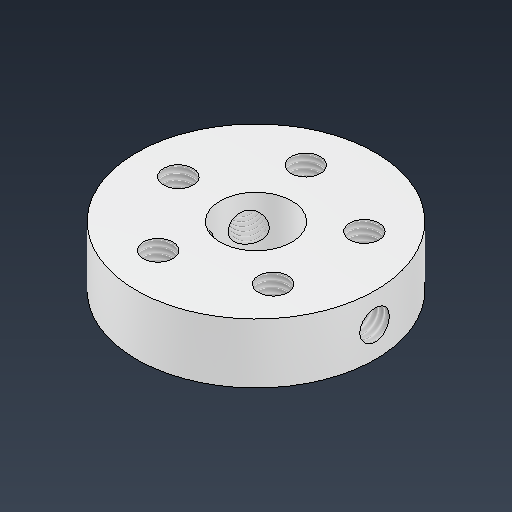
# Autodesk Inventor part: DiyHub
Saved by Autodesk Inventor 2026.2 (Build 302298010, 298A)
## iProperties
Created: 2026-04-20
Part Number: DiyHub
Material: Aluminum 6061
Document SubType Name: Modeling
Designer: szymo
Density: 2.7 g/cm^3
Appearance: Aluminum - Flat
Author: szymo
Autodesk Inventor part; units mm, degrees
ref_plane "YZ Plane" through (0, 0, 0) normal (1, 0, 0) x (0, 1, 0)
ref_plane "XZ Plane" through (0, 0, 0) normal (0, 1, 0) x (-1, 0, 0)
ref_plane "XY Plane" through (0, 0, 0) normal (0, 0, 1) x (1, 0, 0)
sketch "Sketch1" plane through (0, 0, 0) normal (0, 1, 0) x (-1, 0, 0)
  circle A0 centre (0, 0) radius 15 construction
  circle A1 centre (0, 0) radius 10
  circle A2 centre (0, 0) radius 3
  circle A3 centre (0, 0) radius 6.5 construction
  circle A4 centre (6.5, 0) radius 3.25 construction
  line L0 (6.5, 0) -> (0, 0) construction
  circle A5 centre (6.5, 0) radius 1.5 construction
  circle A6 centre (2.0086, 6.1819) radius 1.5 construction
  circle A7 centre (2.0086, 6.1819) radius 3.25 construction
  circle A8 centre (-5.2586, 3.8206) radius 1.5 construction
  circle A9 centre (-5.2586, 3.8206) radius 3.25 construction
  circle A10 centre (-5.2586, -3.8206) radius 1.5 construction
  circle A11 centre (-5.2586, -3.8206) radius 3.25 construction
  circle A12 centre (2.0086, -6.1819) radius 1.5 construction
  circle A13 centre (2.0086, -6.1819) radius 3.25 construction
  dimension "d4" = 13
  dimension "d0" = 30
  dimension "d1" = 5
  dimension "d2" = 20
  dimension "d3" = 6
  dimension "d5" = 6.5
  dimension "d6" = 3
  dimension "d9" = 360
  constraints: 13 centre point, 9 coincident, 2 end point, 1 horizontal, 1 horizontal alignment, 23 other
  measures "d0" diameter of A0
  measures "d1" radial gap between concentric circles of A0 A1
  measures "d2" diameter of A1
  measures "d3" diameter of A2
  measures "d5" diameter of A4
  measures "d6" diameter of A5
extrude "Extrusion1" add sketch "Sketch1" against normal blind 5
hole "Hole1" at (-6.5, 0, 0) at (-2.0086, 0, -6.1819) at (5.2586, 0, -3.8206) at (5.2586, 0, 3.8206) at (-2.0086, 0, 6.1819) direction (0, -1, 0) diameter 2.459 end through all thread size "M3x0.5" class "6H" standard "ISO Metric profile"
sketch "Sketch2" plane through (0, 0, 0) normal (0, 1, 0) x (-1, 0, 0)
  circle A0 centre (0, 0) radius 10
  line L0 (0, 0) -> (-10, 0)
  line L1 (0, 0) -> (8.0902, 5.8779)
  line L2 (0, 0) -> (8.0902, -5.8779)
  circle A1 centre (2.0086, 6.1819) radius 1.2295 projected
  circle A2 centre (2.0086, -6.1819) radius 1.2295 projected
  circle A3 centre (6.5, 0) radius 1.2295 projected
  circle A4 centre (-5.2586, 3.8206) radius 1.2295 projected
  circle A5 centre (-5.2586, -3.8206) radius 1.2295 projected
  dimension "d20" = 20
  dimension "d24" = 3.8206
  dimension "d25" = 3.8206
  dimension "d26" = 3.8206
  dimension "d27" = 3.8206
  constraints: 6 end point, 3 point on circle, 1 centre point, 1 coincident, 1 horizontal
  measures "d20" diameter of A0
  measures "d24" distance from line of L1 A1.centre
  measures "d25" distance from line of A3.centre L1
  measures "d26" distance from line of L2 A3.centre
  measures "d27" distance from line of A2.centre L2
ref_plane "Work Plane1" through (0, 0, 0) normal (-0.809017, 0, 0.5877853) x (0, -1, 0)
ref_plane "Work Plane2" through (0, 0, 0) normal (-0.809017, 0, -0.5877853) x (0, -1, 0)
sketch "Sketch3" plane through (0, 0, 0) normal (1, 0, 0) x (0, 1, 0)
  line L0 (0, 3) -> (0, -3) projected
  line L1 (-5, -3) -> (-5, 3) projected
  line L2 (-5, 3) -> (0, -3)
  line L3 (-5, -3) -> (0, 3)
  point P0 (0, 0)
  point P1 (-2.5, 0)
  constraints: 4 end point, 1 midpoint
hole "Hole2" at (0, -2.5, 0) direction (1, 0, 0) diameter 2.459 depth 20 thread size "M3x0.5" class "6H" standard "ISO Metric profile"
sketch "Sketch4" plane through (0, 0, 0) normal (-0.809017, 0, -0.5877853) x (0, -1, 0)
  line L0 (0, -3) -> (0, 3) projected
  line L1 (5, 3) -> (5, -3) projected
  line L2 (0, -3) -> (5, 3)
  line L3 (5, -3) -> (0, 3)
  point P0 (0, 0)
  point P1 (2.5, 0)
  constraints: 4 end point, 1 midpoint
hole "Hole3" at (0, -2.5, 0) direction (-0.809017, 0, -0.5877853) diameter 2.459 depth 20 thread size "M3x0.5" class "6H" standard "ISO Metric profile"
sketch "Sketch5" plane through (0, 0, 0) normal (-0.809017, 0, 0.5877853) x (0, -1, 0)
  line L0 (0, -3) -> (0, 3) projected
  line L1 (5, 3) -> (5, -3) projected
  line L2 (0, -3) -> (5, 3)
  line L3 (5, -3) -> (0, 3)
  point P0 (0, 0)
  point P1 (2.5, 0)
  constraints: 4 end point, 1 midpoint
hole "Hole4" at (0, -2.5, 0) direction (-0.809017, 0, 0.5877853) diameter 2.459 depth 20 thread size "M3x0.5" class "6H" standard "ISO Metric profile"
equation "\"d24\" = d25"
equation "\"d26\" = d27"
body "Solid1"
